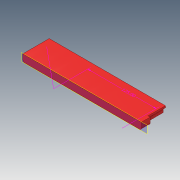
# Autodesk Inventor part: Prova supporti
Saved by Autodesk Inventor 2019 (Build 230136000, 136)
## iProperties
Created: 2019-05-06
Part Number: Prova supporti
Material: Generic
Document SubType Name: Modeling
Designer: giacomo
Density: 1 g/cm^3
Appearance: Light Red
Author: giacomo
Autodesk Inventor part; units mm, degrees
sketch "Sketch1" plane through (0, 0, 0) normal (0, 1, 0) x (-1, 0, 0)
  line L0 (-67.5, 75) -> (67.5, 75)
  line L1 (67.5, 75) -> (67.5, -75)
  line L2 (67.5, -75) -> (-67.5, -75)
  line L3 (-67.5, -75) -> (-67.5, 75)
  line L4 (-67.5, 75) -> (67.5, -75) construction
  line L5 (67.5, 75) -> (-67.5, -75) construction
  point P0 (0, 0)
  dimension "d0" = 135
  dimension "d1" = 150
  constraints: 12 end point, 2 midpoint, 2 parallel, 1 horizontal, 1 perpendicular
  measures "d0" distance of L1.end L2.end
  measures "d1" distance of L0.end L1.end
extrude "Extrusion1" add sketch "Sketch1" along normal blind 8
sketch "Sketch3" plane through (0, 8, 0) normal (0, 1, 0) x (1, 0, 0)
  line L0 (-67.5, -75) -> (67.5, -75) projected
  line L1 (67.5, -75) -> (67.5, 75) projected
  line L2 (67.5, 75) -> (-67.5, 75) projected
  line L3 (-67.5, 75) -> (-67.5, -75) projected
  line L4 (62.5, 75) -> (62.5, -70)
  line L5 (-67.5, -75) -> (67.5, -75) projected
  line L6 (67.5, -75) -> (67.5, 75) projected
  line L7 (0, 0) -> (0, -83) construction
  line L8 (-62.5, 75) -> (-62.5, -70)
  line L9 (62.5, -70) -> (-62.5, -70)
  dimension "d4" = 5
  dimension "d5" = 5
  constraints: 8 end point, 3 parallel, 2 point on line, 1 perpendicular, 1 vertical, 1 other
  measures "d4" distance between parallel lines of L1 L4
  measures "d5" distance between parallel lines of L9 L0
extrude "Extrusion2" add sketch "Sketch3" along normal blind 38.7 contours L3 L2 L8 L9 L4 L1 L0
sketch "Sketch4" plane through (67.5, 0, -75) normal (0, 0, -1) x (-1, 0, 0)
  line L0 (135, 0) -> (0, 0) projected
  line L1 (135, 0) -> (135, 46.7) projected
  line L2 (130, 46.7) -> (135, 46.7) projected
  line L3 (130, 8) -> (130, 46.7) projected
  line L4 (5, 8) -> (130, 8) projected
  line L5 (5, 8) -> (5, 46.7) projected
  line L6 (0, 46.7) -> (5, 46.7) projected
  line L7 (0, 0) -> (0, 46.7) projected
  line L8 (130, 8) -> (5, 8) projected
  line L9 (5, 8) -> (5, 0)
  line L10 (130, 8) -> (130, 0)
  line L11 (0, 0) -> (135, 0) projected
  line L12 (0, 0) -> (0, 46.7) projected
  line L13 (5, 3) -> (130, 3)
  line L14 (5, 8) -> (130, 8) projected
  line L15 (5, 6) -> (130, 6)
  line L16 (5, 8) -> (0, 8)
  line L17 (135, 0) -> (0, 0) projected
  point P0 (67.5, 0)
  dimension "d8" = 3
  dimension "d9" = 3
  constraints: 10 end point, 8 point on line, 6 parallel, 2 perpendicular, 1 vertical
  measures "d8" distance between parallel lines of L0 L13
  measures "d9" distance between parallel lines of L13 L15
extrude "Extrusion3" add sketch "Sketch4" along normal blind 20 contours L0 L10 L3 L2 L1 | L0 L9 L13 L10 | L15 L9 L4 L10 | L7 L6 L5 L16
sketch "Sketch6" plane through (67.5, 0, 75) normal (1, 0, 0) x (0, 0, -1)
  line L0 (150, 0) -> (150, 8)
  line L1 (0, 0) -> (0, 46.7) projected
  line L2 (150, 8) -> (170, 8) projected
  line L3 (0, 46.7) -> (170, 46.7) projected
  line L4 (170, 46.7) -> (170, 8) projected
  line L5 (170, 21) -> (153, 21)
  line L6 (153, 21) -> (153, 33)
  line L7 (153, 33) -> (170, 33)
  line L8 (170, 33) -> (170, 21)
  point P0 (75, 0)
  dimension "d92" = 13
  dimension "d93" = 17
  dimension "d94" = 12
  constraints: 10 end point, 2 parallel, 1 horizontal, 1 perpendicular, 1 point on line
  measures "d92" distance between parallel lines of L2 L5
  measures "d93" distance of L6.end L7.end
  measures "d94" distance of L5.end L6.end
fillet "Fillet1" radius 2 11 edges at (67.5, 0, 0) (67.5, 46.7, -10) (67.5, 23.35, 75) (0, 46.7, 75) (0, 0, 75) (-67.5, 46.7, -10) (-67.5, 23.35, 75) (-67.5, 0, -10) (62.5, 46.7, -12.5) (-62.5, 46.7, -12.5) (0, 46.7, 70)
ref_plane "Work Plane4" through (-67.5, 9.7, -88) normal (-1, 0, 0) x (0, 0, 1)
sketch "Sketch15" plane through (62.5, 6, -75) normal (1, 0, 0) x (0, 0, -1)
  line L0 (0, 0) -> (0, 2) projected
  line L1 (0, 0) -> (20, 0) projected
  line L2 (20, 2) -> (20, 0) projected
  line L3 (0, 2) -> (20, 2) projected
  point P0 (-75, -6)
extrude "Extrusion8" add sketch "Sketch15" along normal blind 2.5
sketch "Sketch16" plane through (0, 8, 0) normal (0, 1, 0) x (1, 0, 0)
  line L0 (-62.5, -35) -> (-46.5, -35)
  line L1 (-46.5, -35) -> (-46.5, 5)
  line L2 (-46.5, 5) -> (-62.5, 5)
  line L3 (-62.5, 5) -> (-62.5, -35)
  line L4 (62.5, -70) -> (-62.5, -70) projected
  line L5 (-62.5, -70) -> (-62.5, 95) projected
  line L6 (46.5, -70) -> (62.5, -70)
  line L7 (62.5, -70) -> (62.5, -30)
  line L8 (62.5, -30) -> (46.5, -30)
  line L9 (46.5, -30) -> (46.5, -70)
  line L10 (62.5, 95) -> (62.5, -70) projected
  point P0 (0, 0)
  dimension "d39" = 35
  dimension "d40" = 0
  dimension "d41" = 16
  dimension "d42" = 40
  dimension "d43" = 0
  dimension "d44" = 0
  dimension "d45" = 40
  dimension "d46" = 16
  constraints: 16 end point, 4 parallel, 2 horizontal, 2 perpendicular
  measures "d39" distance between parallel lines of L4 L0
  measures "d40" distance between parallel lines of L5 L3
  measures "d41" distance between parallel lines of L1 L3
  measures "d42" distance of L0.end L1.end
  measures "d43" distance between parallel lines of L4 L6
  measures "d44" distance between parallel lines of L10 L7
  measures "d45" distance of L8.end L6.start
  measures "d46" distance of L7.end L8.end
extrude "Extrusion9" add sketch "Sketch16" along normal blind 16
fillet "Fillet4" radius 1 8 edges at (46.5, 24, 50) (54.5, 24, 30) (46.5, 16, 30) (-46.5, 24, 15) (-46.5, 16, -5) (-54.5, 24, 35) (-54.5, 24, -5) (-46.5, 16, 35)
sketch "Sketch17" plane through (0, 24, 0) normal (0, 1, 0) x (1, 0, 0)
  circle A0 centre (-56.5, -25) radius 2.25
  line L0 (-62.5, -34) -> (-62.5, 4) projected
  line L1 (-47.5, -34) -> (-62.5, -34) projected
  circle A1 centre (54.5, -57.5) radius 2.25
  line L2 (47.5, -70) -> (47.5, -31) projected
  line L3 (47.5, -31) -> (62.5, -31) projected
  line L4 (62.5, -70) -> (50.5, -70) projected
  point P0 (0, 0)
  dimension "d50" = 4.5
  dimension "d51" = 6
  dimension "d52" = 9
  dimension "d53" = 4.5
  dimension "d54" = 7
  dimension "d90" = 12.5
  constraints: 2 centre point, 1 other
  measures "d50" diameter of A0
  measures "d51" distance from line of L0 A0.centre
  measures "d52" distance from line of L1 A0.centre
  measures "d53" diameter of A1
  measures "d90" distance from line of L4 A1.centre
extrude "Extrusion10" cut sketch "Sketch17" against normal blind 12
ref_plane "Work Plane5" through (-62.5, 9.7, -88) normal (1, 0, 0) x (0, 0, -1)
sketch "Sketch18" plane through (-62.5, 9.7, -88) normal (1, 0, 0) x (0, 0, -1)
  circle A0 centre (-58, 19) radius 2.25
  circle A1 centre (-27.2, 19) radius 2.25
  line L0 (0, 8.1) -> (0, 14.1)
  line L1 (-27.2, 19) -> (-58, 19)
  line L2 (7, 37) -> (-160, 37) projected
  line L3 (-158, -1.7) -> (-158, 35) projected
  point P0 (-88, -9.7)
  dimension "d60" = 4.5
  dimension "d61" = 4.5
  dimension "d62" = 30.8
  dimension "d67" = 100
  dimension "d91" = 18
  constraints: 4 end point, 2 centre point, 1 horizontal
  measures "d60" diameter of A0
  measures "d61" diameter of A1
  measures "d62" distance of L1.start L1.end
  measures "d67" distance from line of L3 L1.end
  measures "d91" distance between parallel lines of L2 L1
extrude "Extrusion11" cut sketch "Sketch18" against normal through all
ref_plane "Work Plane3" through (0, 22.5, 0) normal (0, 1, 0) x (1, 0, 0)
sketch "Sketch21" plane through (0, 22.5, 0) normal (0, 1, 0) x (1, 0, 0)
  circle A0 centre (54.5, -57.5) radius 2.25 projected
  line L0 (50.75, -55.3349) -> (54.5, -53.1699)
  line L1 (54.5, -53.1699) -> (58.25, -55.3349)
  line L2 (58.25, -55.3349) -> (58.25, -59.6651)
  line L3 (58.25, -59.6651) -> (54.5, -61.8301)
  line L4 (54.5, -61.8301) -> (50.75, -59.6651)
  line L5 (50.75, -59.6651) -> (50.75, -55.3349)
  line L6 (-62.5, -35) -> (-62.5, -70) projected
  line L7 (46.5, -70) -> (46.5, -31) projected
  circle A1 centre (-56.5, -25) radius 2.25 projected
  line L8 (-52.75, -27.1651) -> (-56.5, -29.3301)
  line L9 (-56.5, -29.3301) -> (-60.25, -27.1651)
  line L10 (-60.25, -27.1651) -> (-60.25, -22.8349)
  line L11 (-60.25, -22.8349) -> (-56.5, -20.6699)
  line L12 (-56.5, -20.6699) -> (-52.75, -22.8349)
  line L13 (-52.75, -22.8349) -> (-52.75, -27.1651)
  point P0 (0, 0)
  dimension "d78" = 7.5
  dimension "d79" = 7.5
  constraints: 24 end point, 2 coincident, 2 parallel, 26 other
  measures "d78" distance between parallel lines of L2 L5
  measures "d79" distance between parallel lines of L13 L10
extrude "Extrusion13" cut sketch "Sketch21" against normal blind 3.15
extrude "Extrusion14" cut sketch "Sketch6" against normal through all
sketch "Sketch22" plane through (0, 8, 0) normal (0, 1, 0) x (1, 0, 0)
  line L0 (224, -151) -> (-256, -151)
  line L1 (-256, -151) -> (-256, 143)
  line L2 (-256, 143) -> (224, 143)
  line L3 (224, 143) -> (224, -151)
  point P0 (0, 0)
  constraints: 8 end point, 2 parallel, 1 horizontal, 1 perpendicular
extrude "Extrusion15" cut sketch "Sketch22" along normal through all
ref_plane "Work Plane6" through (62.5, 3, -65) normal (0, 0, -1) x (-1, 0, 0)
sketch "Sketch23" plane through (62.5, 3, -65) normal (0, 0, -1) x (-1, 0, 0)
  line L0 (-63, 29) -> (227, 29)
  line L1 (227, 29) -> (227, -39)
  line L2 (227, -39) -> (-63, -39)
  line L3 (-63, -39) -> (-63, 29)
  point P0 (62.5, -3)
  constraints: 8 end point, 2 parallel, 1 horizontal, 1 perpendicular
extrude "Extrusion16" cut sketch "Sketch23" against normal through all
body "Solid1"
